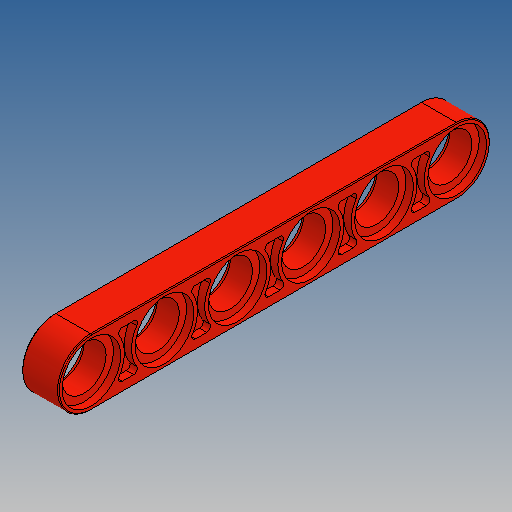
# Autodesk Inventor part: 32063-Red
Saved by Autodesk Inventor 2025 (Build 290162010, 162A)
## iProperties
Created: 2012-03-28
Part Number: 32063-Red
Document SubType Name: Modeling
Designer: D. Kohfeld
Density: 1.06 g/cm^3
Material: ABS Plastic
Mass: 0.751762 g
Surface Area: 13.5862 cm^2
Volume: 0.709209 cm^3
Appearance: Red
Author: D. Kohfeld
Autodesk Inventor part; units mm, degrees
ref_plane "YZ Plane" through (0, 0, 0) normal (1, 0, 0) x (0, 1, 0)
ref_plane "XZ Plane" through (0, 0, 0) normal (0, 1, 0) x (-1, 0, 0)
ref_plane "XY Plane" through (0, 0, 0) normal (0, 0, 1) x (1, 0, 0)
sketch "Sketch3" plane through (0, 0, 0) normal (1, 0, 0) x (0, 1, 0)
  arc A0 (20, -3.6) -> (20, 3.6) centre (20, 0) ccw
  line L0 (-20, -3.6) -> (20, -3.6)
  line L1 (-20, 3.6) -> (20, 3.6)
  arc A1 (-20, 3.6) -> (-20, -3.6) centre (-20, 0) ccw
  line L2 (0, -3.6) -> (0, 3.6) construction
  circle A2 centre (-12, 0) radius 3.2
  circle A3 centre (-4, 0) radius 3.2
  line L3 (-4, 0) -> (-12, 0) construction
  line L4 (-12, 0) -> (-20, 0) construction
  circle A4 centre (-12, 0) radius 2.4
  circle A5 centre (-4, 0) radius 2.4
  circle A6 centre (-20, 0) radius 3.2
  circle A7 centre (-20, 0) radius 2.4
  circle A8 centre (4, 0) radius 3.2
  circle A9 centre (4, 0) radius 2.4
  circle A10 centre (20, 0) radius 3.2
  circle A11 centre (20, 0) radius 2.4
  line L5 (-4, 0) -> (4, 0) construction
  circle A12 centre (12, 0) radius 2.4
  circle A13 centre (12, 0) radius 3.2
  line L6 (4, 0) -> (12, 0) construction
  line L7 (12, 0) -> (20, 0) construction
  point P0 (0, 0)
  point P1 (0, 0)
  dimension "d49" = 7.2
  dimension "d59" = 6.4
  dimension "d60" = 4.8
  dimension "d64" = 8
  constraints: 16 end point, 14 centre point, 10 equal radius, 9 coincident, 5 collinear, 4 equal length, 4 point on circle, 4 tangent, 3 horizontal, 3 midpoint, 1 point on line, 1 symmetric about line
  measures "d49" diameter of A0
  measures "d59" diameter of A2
  measures "d60" diameter of A4
  measures "d64" distance of L5.start L5.end
extrude "Extrusion4" add sketch "Sketch3" along normal mid plane 4 contours L0 A1 L1 A0 | A2 | A3 | A6 | A8 | A10 | A13
sketch "Sketch11" plane through (2, 0, 0) normal (1, 0, 0) x (0, 0, -1)
  circle A0 centre (0, -4) radius 2.4 projected
  circle A1 centre (0, -12) radius 2.4 projected
  circle A2 centre (0, -4) radius 3.2
  circle A3 centre (0, -12) radius 3.2
  circle A4 centre (0, 4) radius 2.4 projected
  arc A5 (3.6, 20) -> (-3.6, 20) centre (0, 20) ccw projected
  arc A6 (-3.6, -20) -> (3.6, -20) centre (0, -20) ccw projected
  circle A7 centre (0, -20) radius 3.2
  circle A8 centre (0, 4) radius 3.2
  circle A9 centre (0, 20) radius 3.2
  circle A10 centre (0, 12) radius 2.4 projected
  circle A11 centre (0, 12) radius 3.2
  circle A12 centre (0, 20) radius 2.4 projected
  line L0 (-3.6, -20) -> (-3.6, 20) projected
  line L1 (-2.5456, 17.4544) -> (-2.5456, 14.5456)
  line L2 (2.5456, 17.4544) -> (2.5456, 14.5456)
  arc A13 (-2.5456, 17.4544) -> (2.5456, 17.4544) centre (0, 20) ccw
  arc A14 (2.5456, 14.5456) -> (-2.5456, 14.5456) centre (0, 12) ccw
  line L3 (-2.5456, 17.4544) -> (0, 20) construction
  line L4 (-2.5456, 9.4544) -> (-2.5456, 6.5456)
  line L5 (2.5456, 9.4544) -> (2.5456, 6.5456)
  arc A15 (-2.5456, 9.4544) -> (2.5456, 9.4544) centre (0, 12) ccw
  arc A16 (2.5456, 6.5456) -> (-2.5456, 6.5456) centre (0, 4) ccw
  line L6 (-2.5456, 1.4544) -> (-2.5456, -1.4544)
  line L7 (2.5456, 1.4544) -> (2.5456, -1.4544)
  arc A17 (-2.5456, 1.4544) -> (2.5456, 1.4544) centre (0, 4) ccw
  arc A18 (2.5456, -1.4544) -> (-2.5456, -1.4544) centre (0, -4) ccw
  line L8 (-2.5456, -6.5456) -> (-2.5456, -9.4544)
  line L9 (2.5456, -6.5456) -> (2.5456, -9.4544)
  arc A19 (-2.5456, -6.5456) -> (2.5456, -6.5456) centre (0, -4) ccw
  arc A20 (2.5456, -9.4544) -> (-2.5456, -9.4544) centre (0, -12) ccw
  line L10 (-2.5456, -14.5456) -> (-2.5456, -17.4544)
  line L11 (2.5456, -14.5456) -> (2.5456, -17.4544)
  arc A21 (-2.5456, -14.5456) -> (2.5456, -14.5456) centre (0, -12) ccw
  arc A22 (2.5456, -17.4544) -> (-2.5456, -17.4544) centre (0, -20) ccw
  point P0 (0, 0)
  dimension "d61" = 6.4
  dimension "d65" = 45
  dimension "d68" = 8
  constraints: 22 end point, 20 point on circle, 16 centre point, 8 coincident, 7 equal radius, 2 parallel, 1 horizontal alignment, 1 vertical, 40 other
  measures "d61" diameter of A3
  measures "d65" angle of L3 L0
  measures "d68" distance of L1.start L4.start
extrude "Extrusion16" cut sketch "Sketch11" against normal blind 0.8 contours A0 | A1 | A2 | A3 | A4 | A7 | A8 | A9 | A10 | A11 | A12
extrude "Extrusion17" cut sketch "Sketch11" against normal blind 0.8 contours A13 L2 A14 L1 | A15 L5 A16 L4 | A17 L7 A18 L6 | A19 L9 A20 L8 | A21 L11 A22 L10
mirror "Mirror3" about plane through (0, 0, 0) normal (1, 0, 0) of "Extrusion16", "Extrusion17"
fillet "Fillet1" radius 0.1 8 edges at (-2, 23.6, 0) (-2, 0, 3.6) (-2, 0, -3.6) (2, 0, 3.6) (2, 0, -3.6) (2, 23.6, 0) (-2, -23.6, 0) (2, -23.6, 0)
fillet "Fillet1" radius 0.4 40 edges at (1.6, -17.4544, 2.5456) (1.6, -14.5456, 2.5456) (1.6, -17.4544, -2.5456) (1.6, -14.5456, -2.5456) (1.6, -9.4544, 2.5456) (1.6, -6.5456, 2.5456) (1.6, -9.4544, -2.5456) (1.6, -6.5456, -2.5456) (1.6, -1.4544, 2.5456) (1.6, -1.4544, -2.5456) (1.6, 1.4544, 2.5456) (1.6, 1.4544, -2.5456) (1.6, 6.5456, 2.5456) (1.6, 6.5456, -2.5456) (1.6, 9.4544, 2.5456) (1.6, 9.4544, -2.5456) (1.6, 14.5456, 2.5456) (1.6, 14.5456, -2.5456) (1.6, 17.4544, 2.5456) (1.6, 17.4544, -2.5456) (-1.6, 17.4544, 2.5456) (-1.6, 14.5456, 2.5456) (-1.6, 17.4544, -2.5456) (-1.6, 14.5456, -2.5456) (-1.6, 9.4544, 2.5456) (-1.6, 6.5456, 2.5456) (-1.6, 9.4544, -2.5456) (-1.6, 6.5456, -2.5456) (-1.6, 1.4544, 2.5456) (-1.6, -1.4544, 2.5456) (-1.6, 1.4544, -2.5456) (-1.6, -1.4544, -2.5456) (-1.6, -6.5456, 2.5456) (-1.6, -6.5456, -2.5456) (-1.6, -9.4544, 2.5456) (-1.6, -9.4544, -2.5456) (-1.6, -14.5456, 2.5456) (-1.6, -14.5456, -2.5456) (-1.6, -17.4544, 2.5456) (-1.6, -17.4544, -2.5456)
equation "\"d49\" = tlad"
equation "\"d59\" = tsd"
equation "\"d60\" = tpd"
equation "\"d64\" = lu"
equation "\"d15\" = 0.5 * lu"
equation "\"d61\" = tsd"
equation "\"d68\" = lu"
equation "\"d62\" = tsl"
equation "\"d73\" = 0.5 * lu - 2 * wall"
equation "\"tlad\" = 7.2"
equation "\"tsd\" = 6.4"
equation "\"tpd\" = 4.8"
equation "\"lu\" = 8"
equation "\"tsl\" = 0.8"
equation "\"wall\" = 1.6"
body "Solid1"
